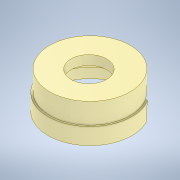
# Autodesk Inventor part: Top of Housing.ipt v2
Saved by Autodesk Inventor 2022 (Build 260153000, 153)
## iProperties
Created: 2023-01-16
Part Number: Top of Housing.ipt v2
Material: Generic
Document SubType Name: Modeling
Designer: ASUS
Density: 1 g/cm^3
Appearance: Nylon 6
Author: ASUS
Autodesk Inventor part; units mm, degrees
ref_plane "YZ Plane" through (0, 0, 0) normal (1, 0, 0) x (0, 1, 0)
ref_plane "XZ Plane" through (0, 0, 0) normal (0, 1, 0) x (-1, 0, 0)
ref_plane "XY Plane" through (0, 0, 0) normal (0, 0, 1) x (1, 0, 0)
sketch "Sketch1" plane through (0, 0, 0) normal (1, 0, 0) x (0, 1, 0)
  line L0 (0, 14.6) -> (6.55, 14.6)
  line L1 (6.55, 14.6) -> (6.55, 16.2)
  line L2 (0, 0) -> (0, 21.161) construction
  line L3 (6.55, 16.2) -> (0, 16.2)
  line L4 (0, 16.2) -> (0, 18.2)
  line L5 (0, 18.2) -> (8.5, 18.2)
  line L6 (8.5, 18.2) -> (8.5, 10.2659) construction
  line L7 (8.5, 13.1) -> (3, 13.1)
  line L8 (8.5, 18.2) -> (8.5, 13.1)
  line L9 (0, 2.5) -> (3, 2.5)
  line L10 (0, 0) -> (11.9587, 0) construction
  line L11 (3, 2.5) -> (3, 13.1)
  line L12 (0, 14.6) -> (0, 2.5)
  line L13 (6.55, 16.2) -> (8.5, 16.2)
  dimension "d0" = 6.55
  dimension "d1" = 14.6
  dimension "d2" = 16.2
  dimension "d3" = 2
  dimension "d4" = 8.5
  dimension "d5" = 1.5
  dimension "d6" = 3
  dimension "d7" = 2.5
  constraints: 28 end point, 8 perpendicular, 6 point on line, 3 horizontal, 2 vertical
  measures "d0" distance of L0.start L0.end
  measures "d1" distance from line of L2.start L0
  measures "d2" vertical distance of L2.start L1.end
  measures "d3" distance of L3.end L4.end
  measures "d4" distance of L4.end L5.end
  measures "d5" distance between parallel lines of L7 L0
  measures "d6" distance of L9.start L9.end
  measures "d7" distance between parallel lines of L10 L9
revolve "Revolution1" add sketch "Sketch1" angle 360 about axis through (0, 0, 0) along (0, 1, 0) contours L3 L4 L5 L8 L13
sketch "Sketch5" plane through (0, 8.5, 0) normal (0, 1, 0) x (1, 0, 0)
  line L0 (0, 0) -> (0, 1)
  circle A0 centre (0, 1) radius 35
  circle A1 centre (0, 1) radius 36.5
  circle A2 centre (0, 0) radius 16.2
  dimension "d29" = 1
  dimension "d30" = 70
  dimension "d31" = 73
  constraints: 3 centre point, 3 coincident, 2 end point, 1 vertical
  measures "d29" distance of L0.start L0.end
  measures "d30" diameter of A0
  measures "d31" diameter of A1
extrude "Extrusion2" add sketch "Sketch5" against normal blind 3 contours A0 | A2
extrude "Extrusion3" add sketch "Sketch5" against normal blind 23.7 contours A1
sketch "Sketch7" plane through (0, 5.5, 0) normal (0, -1, 0) x (1, 0, 0)
  circle A0 centre (0, 0) radius 16.2
  constraints: 1 centre point, 1 coincident
extrude "Extrusion5" cut sketch "Sketch7" against normal blind 10
sketch "Sketch8" plane through (0, -15.2, 0) normal (0, -1, 0) x (1, 0, 0)
  circle A0 centre (0, -1) radius 36.5
  circle A1 centre (0, -1) radius 38
  point P0 (0, 0)
  dimension "d43" = 73
  dimension "d44" = 1
  dimension "d45" = 76
  constraints: 2 centre point, 1 coincident
  measures "d43" diameter of A0
  measures "d44" distance of point (0, 0) A0.centre
  measures "d45" diameter of A1
extrude "Extrusion6" add sketch "Sketch8" along normal blind 10 and the other way blind 5
sketch "Sketch6" plane through (0, 0, 0) normal (1, 0, 0) x (0, 1, 0)
  line L0 (-15.2, -36) -> (-15.2, 34) projected
  line L1 (-15.2, 0) -> (-15.2, -19.5)
  line L2 (-15.2, -19.5) -> (-15.2, -27)
  circle A0 centre (-15.2, -27) radius 7.75
  point P0 (0, 0)
  dimension "d36" = 19.5
  dimension "d37" = 7.5
  dimension "d38" = 15.5
  constraints: 4 end point, 3 point on line, 1 centre point, 1 coincident
  measures "d36" distance of L1.start L1.end
  measures "d37" distance of L1.end L2.end
  measures "d38" diameter of A0
extrude "Extrusion4" cut sketch "Sketch6" along normal through all
sketch "Sketch9" plane through (0, 0, 0) normal (1, 0, 0) x (0, 1, 0)
  line L0 (-15.2, -19.25) -> (-25.2, -19.25)
  line L1 (-25.2, -37.5) -> (-25.2, 35.5) projected
  line L2 (-15.2, -34.75) -> (-25.2, -34.75)
  line L3 (-25.2, -34.75) -> (-25.2, -19.25)
  line L4 (-15.2, -19.25) -> (-15.2, -34.75)
  point P0 (0, 0)
  constraints: 8 end point, 2 horizontal, 1 parallel, 1 perpendicular, 1 point on line
extrude "Extrusion7" cut sketch "Sketch9" along normal through all
sketch "Sketch10" plane through (0, 0, 0) normal (1, 0, 0) x (0, 1, 0)
  line L0 (-15.2, -36) -> (-15.2, 34) projected
  line L1 (-15.2, -0.25) -> (-15.2, -20.75)
  line L2 (-15.2, -20.75) -> (-15.2, -28.25)
  circle A0 centre (-15.2, -28.25) radius 9
  line L3 (-15.2, -19.25) -> (-25.2, -19.25)
  line L4 (-15.2, -37.25) -> (-25.2, -37.25)
  line L5 (-25.2, -37.25) -> (-25.2, -19.25)
  point P0 (0, 0)
  point P1 (-15.2, -34.75)
  point P2 (-15.2, -19.25)
  point P3 (-25.2, -34.75)
  dimension "d57" = 20.5
  dimension "d58" = 7.5
  dimension "d59" = 18
  constraints: 10 end point, 4 point on line, 2 horizontal, 2 point on circle, 1 centre point, 1 coincident, 1 perpendicular, 1 tangent
  measures "d57" distance of L1.start L1.end
  measures "d58" distance of L1.end L2.end
  measures "d59" diameter of A0
extrude "Extrusion8" cut sketch "Sketch10" along normal through all
body "Solid1"
